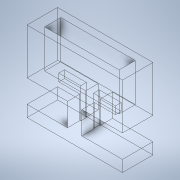
# Autodesk Inventor part: fusebox
Saved by Autodesk Inventor 2021.5 (Build 255421000, 421)
## iProperties
Created: 2025-01-02
Part Number: fusebox
Material: Generic
Document SubType Name: Modeling
Designer: email
Density: 1 g/cm^3
Appearance: Default
Author: email
Autodesk Inventor part; units mm, degrees
ref_plane "YZ Plane" through (0, 0, 0) normal (1, 0, 0) x (0, 1, 0)
ref_plane "XZ Plane" through (0, 0, 0) normal (0, 1, 0) x (-1, 0, 0)
ref_plane "XY Plane" through (0, 0, 0) normal (0, 0, 1) x (1, 0, 0)
sketch "Sketch1" plane through (0, 0, 0) normal (0, 0, 1) x (1, 0, 0)
  line L0 (0, 0) -> (25, 0)
  line L1 (25, 0) -> (25, 12)
  line L2 (25, 12) -> (0, 12)
  line L3 (0, 12) -> (0, 0)
  line L4 (10.625, 0) -> (14.375, 0)
  line L5 (14.375, 0) -> (14.375, -6)
  line L6 (14.375, -6) -> (10.625, -6) construction
  line L7 (10.625, -6) -> (10.625, 0)
  line L8 (0, -6) -> (25, -6)
  line L9 (25, -6) -> (25, -9)
  line L10 (25, -9) -> (0, -9)
  line L11 (0, -9) -> (0, -6)
  point P0 (14.375, 0)
  dimension "d0" = 25
  dimension "d1" = 12
  dimension "d2" = 6
  dimension "d3" = 3.75
  dimension "d4" = 10.625
  dimension "d28" = 0
  dimension "d29" = 3
  constraints: 24 end point, 6 parallel, 3 horizontal, 3 perpendicular, 1 point on line
  measures "d0" distance of L1.end L2.end
  measures "d1" distance of L2.end L0.start
  measures "d2" distance of L4.end L5.end
  measures "d3" distance of L5.end L6.end
  measures "d4" distance between parallel lines of L3 L7
  measures "d28" distance between parallel lines of L6 L8
  measures "d29" distance of L8.end L9.end
extrude "Extrusion1" add sketch "Sketch1" along normal blind 8
sketch "Sketch2" plane through (0, 12, 0) normal (0, 1, 0) x (1, 0, 0)
  line L0 (0, 0) -> (10.625, 0) projected
  line L1 (0, 0) -> (25, 0)
  line L2 (25, 0) -> (25, -8)
  line L3 (25, -8) -> (0, -8)
  line L4 (0, -8) -> (0, 0)
  line L5 (2.75, -1.875) -> (22.25, -1.875)
  line L6 (22.25, -1.875) -> (22.25, -6.125)
  line L7 (22.25, -6.125) -> (2.75, -6.125)
  line L8 (2.75, -6.125) -> (2.75, -1.875)
  line L9 (5.05, -4.75) -> (10.8, -4.75)
  line L10 (10.8, -4.75) -> (10.8, -3.25)
  line L11 (10.8, -3.25) -> (5.05, -3.25)
  line L12 (5.05, -3.25) -> (5.05, -4.75)
  line L13 (14.2, -4.75) -> (19.95, -4.75)
  line L14 (19.95, -4.75) -> (19.95, -3.25)
  line L15 (19.95, -3.25) -> (14.2, -3.25)
  line L16 (14.2, -3.25) -> (14.2, -4.75)
  line L17 (2.95, -6) -> (22.05, -6) construction
  line L18 (22.05, -6) -> (22.05, -2) construction
  line L19 (22.05, -2) -> (2.95, -2) construction
  line L20 (2.95, -2) -> (2.95, -6) construction
  dimension "d7" = 25
  dimension "d8" = 8
  dimension "d9" = 19.5
  dimension "d10" = 4.25
  dimension "d11" = 1.875
  dimension "d12" = 2.75
  dimension "d13" = 1.5
  dimension "d14" = 19.1
  dimension "d15" = 4
  dimension "d16" = 2.95
  dimension "d17" = 2
  dimension "d18" = 2.1
  dimension "d20" = 2.1
  dimension "d21" = 1.25
  dimension "d22" = 5.75
  dimension "d23" = 5.75
  constraints: 40 end point, 10 parallel, 5 horizontal, 5 perpendicular, 2 point on line
  measures "d7" distance of L2.end L3.end
  measures "d8" distance of L1.end L2.end
  measures "d9" distance of L5.start L5.end
  measures "d10" distance of L5.end L6.end
  measures "d11" distance between parallel lines of L0 L5
  measures "d12" distance between parallel lines of L4 L8
  measures "d13" distance of L11.end L9.start
  measures "d14" distance of L18.end L19.end
  measures "d15" distance of L17.end L18.end
  measures "d16" distance between parallel lines of L4 L20
  measures "d17" distance between parallel lines of L3 L17
  measures "d18" distance between parallel lines of L20 L12
  measures "d20" distance between parallel lines of L18 L14
  measures "d21" distance between parallel lines of L19 L11
  measures "d22" distance of L9.start L9.end
  measures "d23" distance of L13.start L13.end
extrude "Extrusion2" cut sketch "Sketch2" against normal blind 10 contours L5 L6 L7 L8 | L12 L11 L10 L9 | L16 L15 L14 L13
extrude "Extrusion3" cut sketch "Sketch2" against normal blind 18 contours L12 L11 L10 L9 | L16 L15 L14 L13
body "Solid1"
